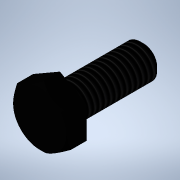
# Autodesk Inventor part: 61581400_5
Saved by Autodesk Inventor 2021 (Build 250183000, 183)
## iProperties
Created: 2026-05-06
Part Number: 61581400_5
Material: Generic
Catalog Web Link: www.3dfindit.com
Description: schr_schrschei_st-Screw, Shrink Disks ST, For very high torques
Vendor: MAEDLER
Document SubType Name: Modeling
Designer: psAdmin
Manufacturer: MAEDLER
Mass: 0.417813 g
Surface Area: 3.84584 cm^2
Volume: 0.417813 cm^3
Density: 1 g/cm^3
Appearance: PSOLRGB-44-44-44
Category: PARTsolutions
Company: MAEDLER
Title: 61581400
Author: Cadenas PARTsolutions
Comments: Screw, Shrink Disks ST, For very high torques
PSOL_IDENT_0: {$CADENAS_DATA/23d-libs/maedler/antriebselemente/spannbuchsen_und_spannsaetze/schrumpfscheiben/schru
PSOL_IDENT_1: mpfscheibe_st/schr_schrschei_st.prj},169 {VTYP=3D},{NB=61581400_5},{LINA=61581400},{NN=schr_schrsche
PSOL_IDENT_2: i_st},{DATE=03.01.2025 08:51:46},{GEOMDATE=03.01.2025 06:34:05},{VERSION=},{LINEID=20},{WBVAR=},{WBN
PSOL_IDENT_3: UMERIC=}  {NB=61581400_5},{LINA=61581400},{KT=DUMMY},{ARTNR=61581400},{WEBSHOP=Produktdetails / Kata
PSOL_IDENT_4: logseite / Montageanleitung},{MATK=Stahl brüniert},{MAT=Hochwertiger Stahl 42CrMo4},{SSG=5},{SSL=12}
PSOL_IDENT_5: ,{K=3.5},{SDW=6.9},{SW=8},{HDW=0.5},{CTN=84839089}
NB: 61581400_5
NN: schr_schrschei_st
NT: Screw, Shrink Disks ST, For very high torques
NBSYN: $ARTNR._5
LINA: 61581400
CATALOG: MÄDLER
ARTNR: 61581400
WEBSHOP: Produktdetails / Katalogseite / Montageanleitung
MATK: Stahl brüniert
MAT: Hochwertiger Stahl 42CrMo4
SSG: 5
SSL: 12
K: 3.5
SDW: 6.9
SW: 8
HDW: 0.5
CTN: 84839089
SUPPLIER: MAEDLER
ARTICLENO: 61581400_5
BOMINFO: 61581400
CREATOR: CADENAS GmbH
Autodesk Inventor part; units mm, degrees
sketch "Sketch_1" plane through (0, 0, 0) normal (0, 0, 1) x (1, 0, 0)
  line L0 (-4, -2.3094) -> (0, -4.6188)
  line L1 (0, -4.6188) -> (4, -2.3094)
  line L2 (4, -2.3094) -> (4, 2.3094)
  line L3 (4, 2.3094) -> (0, 4.6188)
  line L4 (0, 4.6188) -> (-4, 2.3094)
  line L5 (-4, 2.3094) -> (-4, -2.3094)
  constraints: 12 end point
extrude "Extrusion1" add sketch "Sketch_1" against normal blind 3
sketch "Sketch_2" plane through (0, 0, 0) normal (1, 0, 0) x (0, 0, -1)
  line L0 (3.5, 0) -> (3, 0)
  line L1 (3, 0) -> (3, 3.45)
  line L2 (3, 3.45) -> (3.5, 3.45)
  line L3 (3.5, 3.45) -> (3.5, 0)
  line L4 (3.5, 0) -> (3, 0)
  constraints: 10 end point
revolve "Revolution1" add sketch "Sketch_2" angle 360 about axis through (0, 0, -3.5) along (0, 0, -1)
sketch "Sketch_3" plane through (0, 0, 0) normal (1, 0, 0) x (0, 0, -1)
  line L0 (15.5, 0) -> (3.5, 0)
  line L1 (3.5, 0) -> (3.5, 2.5)
  line L2 (3.5, 2.5) -> (15.0095, 2.5)
  line L3 (15.0095, 2.5) -> (15.5, 2.0095)
  line L4 (15.5, 2.0095) -> (15.5, 0)
  line L5 (15.5, 0) -> (3.5, 0)
  constraints: 12 end point
revolve "Revolution2" add sketch "Sketch_3" angle 360 about axis through (0, 0, -15.5) along (0, 0, -1)
thread "Thread1" size "M5x0.8" class "6g" standard "ISO Metric profile" full length
sketch "Sketch_4" plane through (0, 0, 0) normal (1, 0, 0) x (0, 0, -1)
  line L0 (50, 0) -> (-50, 0)
  line L1 (-2, 3.9903) -> (0, 3.9903)
  line L2 (0, 3.9903) -> (0.6285, 4.6188)
  line L3 (0.6285, 4.6188) -> (0.6285, 6.6188)
  line L4 (0.6285, 6.6188) -> (-2, 6.6188)
  line L5 (-2, 6.6188) -> (-2, 3.9903)
  constraints: 12 end point
revolve "Revolution3" cut sketch "Sketch_4" angle 360 about axis through (0, 0, -50) along (0, 0, -1)
ref_plane "schraube_st_XY" through (0, 0, -3.5) normal (0, 0, 1) x (1, 0, 0)
ref_plane "schraube_st_YZ" through (0, 0, -3.5) normal (1, 0, 0) x (0, 1, 0)
ref_plane "schraube_st_ZX" through (0, 0, -3.5) normal (0, 1, 0) x (0, 0, 1)
body "Solid1"
